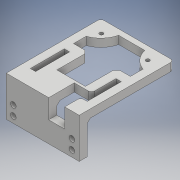
# Autodesk Inventor part: OpenMVMount-Tate-Shortv2
Saved by Autodesk Inventor 2018.3 (Build 223284000, 284)
## iProperties
Created: 2019-04-14
Part Number: OpenMVMount-Tate-Shortv2
Material: 一般
Document SubType Name: Modeling
Designer: shun2
Density: 1 g/cm^3
Appearance: 既定
Author: shun2
Autodesk Inventor part; units mm, degrees
ref_plane "YZ Plane" through (0, 0, 0) normal (1, 0, 0) x (0, 1, 0)
ref_plane "XZ Plane" through (0, 0, 0) normal (0, 1, 0) x (-1, 0, 0)
ref_plane "XY Plane" through (0, 0, 0) normal (0, 0, 1) x (1, 0, 0)
sketch "スケッチ1" plane through (0, 0, 0) normal (0, 0, 1) x (1, 0, 0)
  arc A0 (9.78, 38.045) -> (9.78, 34.091) centre (7.803, 36.068) ccw
  line L0 (9.78, 38.045) -> (9.78, 44.068)
  line L1 (9.78, 28.068) -> (9.78, 34.091)
  line L2 (25.78, 28.068) -> (9.78, 28.068)
  line L3 (25.78, 34.091) -> (25.78, 28.068)
  arc A1 (25.78, 34.091) -> (25.78, 38.045) centre (27.757, 36.068) ccw
  line L4 (25.78, 44.068) -> (25.78, 38.045)
  line L5 (9.78, 44.068) -> (25.78, 44.068)
  line L6 (-3, 49.068) -> (38.56, 49.068)
  line L7 (-5, -5) -> (-5, 47.068)
  arc A2 (0, 34.9259) -> (9.5946, 45.6044) centre (-5, 49.068) ccw
  line L8 (9.5946, 45.6044) -> (25.9654, 45.6044)
  line L9 (0, 21.31) -> (3.3, 21.31)
  line L10 (3.3, 21.31) -> (3.3, 0)
  line L11 (35.56, 21.31) -> (32.26, 21.31)
  line L12 (32.26, 21.31) -> (32.26, 8)
  line L13 (21.5, -5) -> (21.5, 6)
  line L14 (21.5, 6) -> (30.26, 6)
  arc A3 (25.9654, 45.6044) -> (35.56, 34.9259) centre (40.56, 49.068) ccw
  line L15 (9.0644, 24.9241) -> (26.8895, 24.9241)
  line L16 (26.8895, 24.9241) -> (26.8895, 7.5355)
  line L17 (26.8895, 7.5355) -> (9.0644, 7.5355)
  line L18 (9.0644, 7.5355) -> (9.0644, 24.9241)
  line L19 (9.0644, 24.9241) -> (6.9885, 27)
  line L20 (9.0644, 24.9241) -> (12.0002, 24.9241) construction
  line L21 (26.8895, 24.9241) -> (28.9655, 27)
  line L22 (26.8895, 24.9241) -> (29.8253, 24.9241) construction
  line L23 (35.56, 27) -> (28.9655, 27)
  line L24 (6.9885, 27) -> (0, 27)
  line L25 (0, 34.9259) -> (0, 27)
  line L26 (0, 21.31) -> (0, 0)
  line L27 (35.56, 34.9259) -> (35.56, 27)
  line L28 (35.56, 21.31) -> (35.56, 0)
  line L29 (35.56, 0) -> (33.5, 0)
  line L30 (3.3, 0) -> (0, 0)
  arc A4 (-3, 49.068) -> (-5, 47.068) centre (-3, 47.068) ccw
  arc A5 (40.56, 47.068) -> (38.56, 49.068) centre (38.56, 47.068) ccw
  line L31 (-5, -10) -> (-5, -5)
  line L32 (21.5, -10) -> (21.5, -5)
  circle A6 centre (3.302, 41.148) radius 1.15
  circle A7 centre (32.258, 41.148) radius 1.15
  line L33 (40.56, 47.068) -> (40.56, -10)
  line L34 (31.5, -10) -> (31.5, -2)
  arc A8 (30.26, 6) -> (32.26, 8) centre (30.26, 8) ccw
  arc A9 (33.5, 0) -> (31.5, -2) centre (33.5, -2) ccw
  line L35 (-5, -10) -> (21.5, -10)
  line L36 (31.5, -10) -> (40.56, -10)
  dimension "d0" = 3.3
  dimension "d1" = 3.3
  dimension "d2" = 135
  dimension "d3" = 45
  dimension "d4" = 2
  dimension "d5" = 2.3
  dimension "d6" = 2.3
  dimension "d7" = 2
  dimension "d8" = 2
  constraints: 74 end point, 16 point on circle, 10 centre point, 8 perpendicular, 7 horizontal, 5 point on line, 5 tangent, 4 coincident, 3 parallel, 2 equal length, 1 collinear, 1 equal radius, 1 vertical
  measures "d0" distance of L26.start L10.start
  measures "d1" distance of L28.start L12.start
  measures "d2" angle of L20 L19
  measures "d3" angle of L22 L21
  measures "d4" radius of A4
  measures "d5" diameter of A6
  measures "d6" diameter of A7
  measures "d7" radius of A8
  measures "d8" radius of A9
extrude "押し出し1" add sketch "スケッチ1" along normal blind 5 contours L6 A5 L33 L36 L34 A9 L29 L28 L11 L12 A8 L14 L13 L32 L35 L31 L7 A4
sketch "スケッチ2" plane through (0, 0, 0) normal (0, 0, -1) x (-1, 0, 0)
  arc A0 (-38.56, 49.068) -> (-40.56, 47.068) centre (-38.56, 47.068) ccw projected
  line L0 (-40.56, -10) -> (-40.56, 47.068) projected
  line L1 (-31.5, -10) -> (-40.56, -10) projected
  line L2 (-31.5, -2) -> (-31.5, -10) projected
  arc A1 (-31.5, -2) -> (-33.5, 0) centre (-33.5, -2) ccw projected
  line L3 (-35.56, 0) -> (-33.5, 0) projected
  line L4 (-35.56, 21.31) -> (-35.56, 0) projected
  line L5 (-32.26, 21.31) -> (-35.56, 21.31) projected
  line L6 (-32.26, 8) -> (-32.26, 21.31) projected
  arc A2 (-32.26, 8) -> (-30.26, 6) centre (-30.26, 8) ccw projected
  line L7 (-21.5, 6) -> (-30.26, 6) projected
  line L8 (-21.5, -10) -> (-21.5, 6) projected
  line L9 (5, -10) -> (-21.5, -10) projected
  line L10 (5, 47.068) -> (5, -10) projected
  arc A3 (5, 47.068) -> (3, 49.068) centre (3, 47.068) ccw projected
  line L11 (-38.56, 49.068) -> (3, 49.068) projected
  circle A4 centre (-3.302, 41.148) radius 1.15 projected
  circle A5 centre (-32.258, 41.148) radius 1.15 projected
  line L12 (0, 0) -> (-3.3, 0) projected
  line L13 (-3.3, 0) -> (-3.3, 21.31) projected
  line L14 (-3.3, 21.31) -> (0, 21.31) projected
  line L15 (0, 21.31) -> (0, 0) projected
  line L16 (-26.8895, 24.9241) -> (-28.9655, 27) projected
  line L17 (-28.9655, 27) -> (-35.56, 27) projected
  line L18 (-35.56, 27) -> (-35.56, 34.9259) projected
  arc A6 (-35.56, 34.9259) -> (-25.9654, 45.6044) centre (-40.56, 49.068) ccw projected
  line L19 (-25.9654, 45.6044) -> (-9.5946, 45.6044) projected
  arc A7 (-9.5946, 45.6044) -> (0, 34.9259) centre (5, 49.068) ccw projected
  line L20 (0, 34.9259) -> (0, 27) projected
  line L21 (0, 27) -> (-6.9885, 27) projected
  line L22 (-6.9885, 27) -> (-9.0644, 24.9241) projected
  line L23 (-9.0644, 24.9241) -> (-9.0644, 7.5355) projected
  line L24 (-9.0644, 7.5355) -> (-26.8895, 7.5355) projected
  line L25 (-26.8895, 7.5355) -> (-26.8895, 24.9241) projected
  line L26 (5, -10) -> (-40.56, -10)
  line L27 (-40.56, -10) -> (-40.56, -5)
  line L28 (-40.56, -5) -> (5, -5)
  line L29 (5, -5) -> (5, -10)
  dimension "d11" = 5
  constraints: 8 end point, 2 parallel, 1 horizontal, 1 perpendicular, 1 point on line
  measures "d11" distance of L26.end L27.end
extrude "押し出し2" add sketch "スケッチ2" along normal blind 20 contours L28 L2 L1 L0 | L28 L8 L26 L2 | L10 L9 L8 L28
sketch "スケッチ3" plane through (-5, -10, 5) normal (0, -1, 0) x (1, 0, 0)
  circle A0 centre (4.434, -15) radius 1.75
  circle A1 centre (41.06, -21) radius 1.75
  circle A2 centre (4.434, -21) radius 1.75
  circle A3 centre (41.06, -15) radius 1.75
  line L0 (-0.066, -25) -> (-0.066, 0)
  line L1 (45.56, -25) -> (-0.066, -25)
  line L2 (45.56, -25) -> (45.56, 0)
  line L3 (36.5, 0) -> (45.56, 0)
  line L4 (45.56, 0) -> (36.5, 0)
  line L5 (36.5, 0) -> (36.5, -12)
  line L6 (0, 0) -> (26.5, 0)
  line L7 (26.5, 0) -> (26.5, -12)
  line L8 (0, 0) -> (26.5, 0)
  line L9 (45.56, 0) -> (45.56, -25)
  line L10 (36.5, 0) -> (45.56, 0)
  line L11 (36.5, -5) -> (36.5, 0)
  line L12 (26.5, -5) -> (36.5, -5)
  line L13 (26.5, -5) -> (26.5, 0)
  line L14 (0, 0) -> (26.5, 0)
  line L15 (0, 0) -> (0, -25)
  line L16 (45.56, -25) -> (0, -25)
  line L17 (36.5, -12) -> (26.5, -12)
  line L18 (26.5, -12) -> (26.5, -5)
  line L19 (26.5, -5) -> (36.5, -5)
  line L20 (36.5, -5) -> (36.5, -12)
  point P0 (5, -5)
  point P1 (5, -5)
  point P2 (21.3541, -5)
  constraints: 42 end point, 4 centre point, 3 equal length, 2 horizontal, 2 perpendicular
extrude "押し出し3" cut sketch "スケッチ3" against normal blind 20 contours A0 | A1 | A2 | A3 | L5 L17 L7 L12
chamfer "面取り1" distance 2 angle 45 2 edges at (36.03, -5, 0) (8.25, -5, 0)
